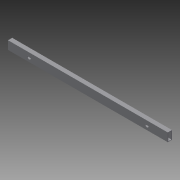
# Autodesk Inventor part: Component 2
Saved by Autodesk Inventor 2015 (Build 190159000, 159)
## iProperties
Created: 2015-01-14
Part Number: Component 2
Material: Generic
Document SubType Name: Modeling
Designer: chapale16
Density: 1 g/cm^3
Appearance: Default
Author: chapale16
Autodesk Inventor part; units mm, degrees
ref_plane "YZ Plane" through (0, 0, 0) normal (1, 0, 0) x (0, 1, 0)
ref_plane "XZ Plane" through (0, 0, 0) normal (0, 1, 0) x (-1, 0, 0)
ref_plane "XY Plane" through (0, 0, 0) normal (0, 0, 1) x (1, 0, 0)
sketch "Sketch1" plane through (0, 0, 0) normal (0, 0, 1) x (1, 0, 0)
  line L0 (0, 0) -> (-965.2, 0)
  line L1 (-965.2, 0) -> (-965.2, 50.8)
  line L2 (-965.2, 50.8) -> (0, 50.8)
  line L3 (0, 50.8) -> (0, 0)
  dimension "d0" = 50.8
  dimension "d1" = 965.2
  constraints: 8 end point, 2 parallel, 1 horizontal, 1 perpendicular
  measures "d0" distance of L2.end L0.start
  measures "d1" distance of L0.start L0.end
extrude "Extrusion1" add sketch "Sketch1" along normal blind 25.4
sketch "Sketch2" plane through (0, 0, 0) normal (1, 0, 0) x (0, 0, -1)
  line L0 (-3.175, 3.175) -> (-22.225, 3.175)
  line L1 (-22.225, 3.175) -> (-22.225, 47.625)
  line L2 (-22.225, 47.625) -> (-3.175, 47.625)
  line L3 (-3.175, 47.625) -> (-3.175, 3.175)
  line L4 (0, 0) -> (-25.4, 0) projected
  line L5 (0, 50.8) -> (0, 0) projected
  line L6 (0, 50.8) -> (-25.4, 50.8) projected
  line L7 (-25.4, 0) -> (-25.4, 50.8) projected
  dimension "d5" = 3.175
  dimension "d7" = 3.175
  dimension "d8" = 3.175
  dimension "d9" = 3.175
  constraints: 8 end point, 2 parallel, 1 horizontal, 1 perpendicular
  measures "d5" distance between parallel lines of L4 L0
  measures "d7" distance between parallel lines of L5 L3
  measures "d8" distance between parallel lines of L6 L2
  measures "d9" distance between parallel lines of L7 L1
extrude "Extrusion2" cut sketch "Sketch2" against normal blind 965.2 contours L0 L1 L2 L3
sketch "Sketch3" plane through (0, 0, 25.4) normal (0, 0, 1) x (1, 0, 0)
  circle A0 centre (-838.2, 25.4) radius 6.2992
  line L0 (-965.2, 0) -> (0, 0)
  line L1 (-965.2, 0) -> (0, 0) projected
  line L2 (-965.2, 50.8) -> (-965.2, 0) projected
  line L3 (0, 0) -> (0, 50.8) projected
  circle A1 centre (-127, 25.4) radius 11.1125
  dimension "d13" = 25.4
  dimension "d14" = 12.5984
  dimension "d16" = 127
  dimension "d18" = 22.225
  constraints: 2 centre point, 2 end point, 1 collinear
  measures "d13" distance from line of L0 A0.centre
  measures "d14" diameter of A0
  measures "d16" distance from line of L2 A0.centre
  measures "d18" diameter of A1
hole "Hole1" at (-838.2, 25.4, 25.4) at (-127, 25.4, 25.4) direction (0, 0, -1) diameter 22.225 end through all
sketch "Sketch4" plane through (0, 0, 0) normal (0, 0, -1) x (-1, 0, 0)
  circle A0 centre (165.735, 38.2537) radius 5.5563 projected
  arc A1 (85.416, 33.4832) -> (85.0155, 42.761) centre (88.5446, 38.2658) ccw projected
  circle A2 centre (165.735, 38.2537) radius 5.5563
  circle A3 centre (88.265, 38.2537) radius 5.5565
  circle A4 centre (88.265, 38.2537) radius 5.5565 projected
  point P0 (0, 0)
  constraints: 2 centre point, 1 coincident, 1 concentric
extrude "Extrusion3" cut sketch "Sketch4" against normal blind 5.08 contours A0 | A3
body "Solid1"
